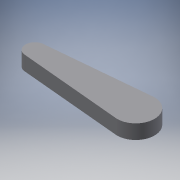
# Autodesk Inventor part: Деталь1
Saved by Autodesk Inventor 2018.3 (Build 223284000, 284)
## iProperties
Created: 2018-06-13
Part Number: Деталь1
Material: Типовые
Document SubType Name: Modeling
Designer: Leancher
Density: 1 g/cm^3
Appearance: По умолчанию
Author: Leancher
Autodesk Inventor part; units mm, degrees
ref_plane "YZ Plane" through (0, 0, 0) normal (1, 0, 0) x (0, 1, 0)
ref_plane "XZ Plane" through (0, 0, 0) normal (0, 1, 0) x (-1, 0, 0)
ref_plane "XY Plane" through (0, 0, 0) normal (0, 0, 1) x (1, 0, 0)
sketch "Эскиз1" plane through (0, 0, 0) normal (0, 0, 1) x (1, 0, 0)
  arc A0 (67.6064, -12.7777) -> (67.6064, 12.7777) centre (70, 0) ccw
  line L0 (0, 6.5) -> (70, 13)
  line L1 (0, -6.5) -> (70, -13)
  arc A1 (0, 6.5) -> (0, -6.5) centre (0, 0) ccw
  dimension "d2" = 26
  constraints: 6 point on circle, 4 end point, 2 centre point, 2 point on line
  measures "d2" diameter of A0
extrude "Выдавливание1" add sketch "Эскиз1" along normal blind 10 contours L1 A1 L0 A0
